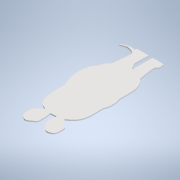
# Autodesk Inventor part: 00Mousetop
Saved by Autodesk Inventor 2022 (Build 260153000, 153)
## iProperties
Created: 2021-10-26
Part Number: 00Mousetop
Material: Generic
Document SubType Name: Modeling
Designer: diederichbenedict
Density: 1 g/cm^3
Appearance: Default
Author: diederichbenedict
Autodesk Inventor part; units mm, degrees
ref_plane "YZ Plane" through (0, 0, 0) normal (1, 0, 0) x (0, 1, 0)
ref_plane "XZ Plane" through (0, 0, 0) normal (0, 1, 0) x (-1, 0, 0)
ref_plane "XY Plane" through (0, 0, 0) normal (0, 0, 1) x (1, 0, 0)
sketch "Sketch1" plane through (0, 0, 0) normal (0, 1, 0) x (-1, 0, 0)
  line L0 (0, 0) -> (305.3292, 0) construction
  line L1 (305.3292, 0) -> (305.3292, -305.3292) construction
  line L2 (305.3292, -305.3292) -> (0, -305.3292) construction
  line L3 (0, -305.3292) -> (0, 0) construction
  line L4 (197.3437, -128.1684) -> (205.2213, -146.037) construction
  line L5 (205.2213, -146.037) -> (209.2562, -163.1371) construction
  line L6 (209.2562, -163.1371) -> (211.1775, -175.8181) construction
  line L7 (211.1775, -175.8181) -> (208.8719, -188.8833) construction
  line L8 (208.8719, -188.8833) -> (206.182, -204.062) construction
  line L9 (206.182, -204.062) -> (200.0285, -210.0785) construction
  line L10 (200.0285, -210.0785) -> (198.478, -210.8805) construction
  line L11 (198.478, -210.8805) -> (195.2992, -224.2295) construction
  line L12 (195.2992, -224.2295) -> (191.0929, -229.9653) construction
  line L13 (191.0929, -229.9653) -> (185.2933, -234.7451) construction
  line L14 (185.2933, -234.7451) -> (185.2933, -235.956) construction
  line L15 (185.2933, -235.956) -> (181.0233, -279.8669) construction
  line L16 (181.0233, -279.8669) -> (181.0233, -282.926) construction
  line L17 (181.0233, -282.926) -> (187.269, -287.196) construction
  line L18 (187.269, -287.196) -> (201.7997, -291.1473) construction
  line L19 (201.7997, -291.1473) -> (205.4962, -289.9364) construction
  line L20 (205.4962, -289.9364) -> (216.5217, -285.7939) construction
  line L21 (216.5217, -285.7939) -> (217.4139, -283.7545) construction
  line L22 (217.4139, -283.7545) -> (218.3315, -284.4307) construction
  line L23 (218.3315, -284.4307) -> (217.6576, -286.08) construction
  line L24 (217.6576, -286.08) -> (211.7874, -290.7265) construction
  line L25 (211.7874, -290.7265) -> (204.5517, -293.4931) construction
  line L26 (204.5517, -293.4931) -> (199.6393, -294.5926) construction
  line L27 (199.6393, -294.5926) -> (192.3503, -294.5926) construction
  line L28 (192.3503, -294.5926) -> (187.225, -293.4044) construction
  line L29 (187.225, -293.4044) -> (186.6398, -292.7482) construction
  line L30 (186.6398, -292.7482) -> (185.9127, -297.8735) construction
  line L31 (185.9127, -297.8735) -> (185.9127, -298.272) construction
  line L32 (185.9127, -298.272) -> (156.9203, -298.272) construction
  line L33 (156.9203, -298.272) -> (156.4747, -298.1064) construction
  line L34 (156.4747, -298.1064) -> (156.4747, -298.9271) construction
  line L35 (156.4747, -298.9271) -> (157.4641, -264.6155) construction
  line L36 (157.4641, -264.6155) -> (157.4641, -263.3694) construction
  line L37 (157.4641, -263.3694) -> (146.4157, -245.343) construction
  line L38 (146.4157, -245.343) -> (146.6138, -244.6411) construction
  line L39 (146.6138, -244.6411) -> (146.902, -296.509) construction
  line L40 (146.902, -296.509) -> (146.902, -298.1341) construction
  line L41 (146.902, -298.1341) -> (145.3394, -298.4778) construction
  line L42 (145.3394, -298.4778) -> (118.2755, -298.1966) construction
  line L43 (118.2755, -298.1966) -> (118.2755, -297.759) construction
  line L44 (118.2755, -297.759) -> (118.2755, -296.9465) construction
  line L45 (118.2755, -296.9465) -> (116.9941, -287.7585) construction
  line L46 (116.9941, -287.7585) -> (116.9941, -285.4771) construction
  line L47 (116.9941, -285.4771) -> (122.6194, -279.1956) construction
  line L48 (122.6194, -279.1956) -> (123.9945, -277.9142) construction
  line L49 (123.9945, -277.9142) -> (117.0254, -237.8184) construction
  line L50 (117.0254, -237.8184) -> (117.0254, -237.0058) construction
  line L51 (117.0254, -237.0058) -> (113.2752, -234.4119) construction
  line L52 (113.2752, -234.4119) -> (107.3686, -227.4741) construction
  line L53 (107.3686, -227.4741) -> (102.0871, -218.2861) construction
  line L54 (102.0871, -218.2861) -> (98.7744, -202.5978) construction
  line L55 (98.7744, -202.5978) -> (99.1182, -169.721) construction
  line L56 (99.1182, -169.721) -> (99.3995, -168.2522) construction
  line L57 (99.3995, -168.2522) -> (98.5869, -167.4397) construction
  line L58 (98.5869, -167.4397) -> (95.3367, -156.9391) construction
  line L59 (95.3367, -156.9391) -> (94.8992, -140.5945) construction
  line L60 (94.8992, -140.5945) -> (97.1806, -133.0316) construction
  line L61 (97.1806, -133.0316) -> (99.6495, -126.7813) construction
  line L62 (99.6495, -126.7813) -> (99.6495, -126.3125) construction
  line L63 (99.6495, -126.3125) -> (98.2431, -95.4359) construction
  line L64 (98.2431, -95.4359) -> (101.2121, -79.5913) construction
  line L65 (101.2121, -79.5913) -> (109.4937, -64.403) construction
  line L66 (109.4937, -64.403) -> (125.2758, -55.6838) construction
  line L67 (125.2758, -55.6838) -> (123.7132, -54.715) construction
  line L68 (123.7132, -54.715) -> (121.9319, -53.6524) construction
  line L69 (121.9319, -53.6524) -> (103.5247, -36.9328) construction
  line L70 (103.5247, -36.9328) -> (103.5247, -35.4015) construction
  line L71 (103.5247, -35.4015) -> (103.9934, -17.1505) construction
  line L72 (103.9934, -17.1505) -> (105.6498, -11.4002) construction
  line L73 (105.6498, -11.4002) -> (115.1503, -7.9) construction
  line L74 (115.1503, -7.9) -> (123.2132, -4.8686) construction
  line L75 (123.2132, -4.8686) -> (135.3701, -19.5881) construction
  line L76 (135.3701, -19.5881) -> (140.6204, -23.5571) construction
  line L77 (140.6204, -23.5571) -> (141.4329, -32.8701) construction
  line L78 (141.4329, -32.8701) -> (138.9015, -52.7461) construction
  line L79 (138.9015, -52.7461) -> (140.5266, -51.9023) construction
  line L80 (140.5266, -51.9023) -> (151.1834, -50.5898) construction
  line L81 (151.1834, -50.5898) -> (155.7149, -51.0898) construction
  line L82 (155.7149, -51.0898) -> (154.6211, -49.5897) construction
  line L83 (154.6211, -49.5897) -> (152.0272, -39.1829) construction
  line L84 (152.0272, -39.1829) -> (152.6646, -20.1194) construction
  line L85 (152.6646, -20.1194) -> (152.6646, -17.1505) construction
  line L86 (152.6646, -17.1505) -> (169.8094, -5.2124) construction
  line L87 (169.8094, -5.2124) -> (175.1222, -4.6498) construction
  line L88 (175.1222, -4.6498) -> (185.8415, -13.3066) construction
  line L89 (185.8415, -13.3066) -> (187.3728, -16.5567) construction
  line L90 (187.3728, -16.5567) -> (187.9979, -36.1828) construction
  line L91 (187.9979, -36.1828) -> (188.2791, -38.7454) construction
  line L92 (188.2791, -38.7454) -> (170.8407, -53.0586) construction
  line L93 (170.8407, -53.0586) -> (169.0906, -53.8712) construction
  line L94 (169.0906, -53.8712) -> (176.2785, -56.2151) construction
  line L95 (176.2785, -56.2151) -> (189.4081, -62.0568) construction
  line L96 (189.4081, -62.0568) -> (195.9358, -82.2789) construction
  line L97 (195.9358, -82.2789) -> (197.3437, -94.6546) construction
  line L98 (197.3437, -94.6546) -> (197.9671, -108.8116) construction
  line L99 (197.9671, -108.8116) -> (197.3437, -128.1684) construction
  spline S0 degree 4 poles (197.3437, -128.1684) (205.2213, -146.037) (209.2562, -163.1371) (211.1775, -175.8181) (208.8719, -188.8833) (206.182, -204.062) (200.0285, -210.0785) (198.478, -210.8805) (195.2992, -224.2295) (191.0929, -229.9653) (185.2933, -234.7451) (185.2933, -235.956) (181.0233, -279.8669) (181.0233, -282.926) (187.269, -287.196) (201.7997, -291.1473) (205.4962, -289.9364) (216.5217, -285.7939) (217.4139, -283.7545) (218.3315, -284.4307) (217.6576, -286.08) (211.7874, -290.7265) (204.5517, -293.4931) (199.6393, -294.5926) (192.3503, -294.5926) (187.225, -293.4044) (186.6398, -292.7482) (185.9127, -297.8735) (185.9127, -298.272) (156.9203, -298.272) (156.4747, -298.1064) (156.4747, -298.9271) (157.4641, -264.6155) (157.4641, -263.3694) (146.4157, -245.343) (146.6138, -244.6411) (146.902, -296.509) (146.902, -298.1341) (145.3394, -298.4778) (118.2755, -298.1966) (118.2755, -297.759) (118.2755, -296.9465) (116.9941, -287.7585) (116.9941, -285.4771) (122.6194, -279.1956) (123.9945, -277.9142) (117.0254, -237.8184) (117.0254, -237.0058) (113.2752, -234.4119) (107.3686, -227.4741) (102.0871, -218.2861) (98.7744, -202.5978) (99.1182, -169.721) (99.3995, -168.2522) (98.5869, -167.4397) (95.3367, -156.9391) (94.8992, -140.5945) (97.1806, -133.0316) (99.6495, -126.7813) (99.6495, -126.3125) (98.2431, -95.4359) (101.2121, -79.5913) (109.4937, -64.403) (125.2758, -55.6838) (123.7132, -54.715) (121.9319, -53.6524) (103.5247, -36.9328) (103.5247, -35.4015) (103.9934, -17.1505) (105.6498, -11.4002) (115.1503, -7.9) (123.2132, -4.8686) (135.3701, -19.5881) (140.6204, -23.5571) (141.4329, -32.8701) (138.9015, -52.7461) (140.5266, -51.9023) (151.1834, -50.5898) (155.7149, -51.0898) (154.6211, -49.5897) (152.0272, -39.1829) (152.6646, -20.1194) (152.6646, -17.1505) (169.8094, -5.2124) (175.1222, -4.6498) (185.8415, -13.3066) (187.3728, -16.5567) (187.9979, -36.1828) (188.2791, -38.7454) (170.8407, -53.0586) (169.0906, -53.8712) (176.2785, -56.2151) (189.4081, -62.0568) (195.9358, -82.2789) (197.3437, -94.6546) (197.9671, -108.8116) (197.3437, -128.1684) knots 1 1 1 1 1 2 3 4 5 6 7 8 9 10 11 12 13 14 15 16 17 18 19 20 21 22 23 24 25 26 27 28 29 30 31 32 33 34 35 36 37 38 39 40 41 42 43 44 45 46 47 48 49 50 51 52 53 54 55 56 57 58 59 60 61 62 63 64 65 66 67 68 69 70 71 72 73 74 75 76 77 78 79 80 81 82 83 84 85 86 87 88 89 90 91 92 93 94 94 94 94 94
  constraints: 13 vertical, 2 horizontal, 3 other
extrude "Extrusion1" add sketch "Sketch1" along normal blind 3
body "Solid1"
